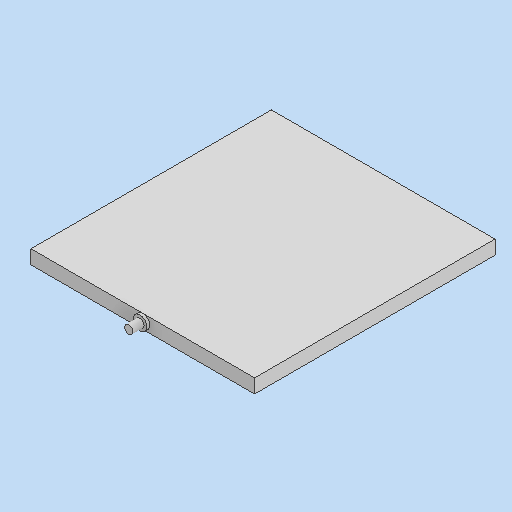
# Autodesk Inventor part: brush
Saved by Autodesk Inventor 2026 (Build 300175000, 175)
## iProperties
Created: 2026-02-15
Part Number: brush
Material: Generic
Document SubType Name: Modeling
Designer: mones
Density: 1 g/cm^3
Appearance: Default
Author: mones
Autodesk Inventor part; units mm, degrees
ref_plane "YZ Plane" through (0, 0, 0) normal (1, 0, 0) x (0, 1, 0)
ref_plane "XZ Plane" through (0, 0, 0) normal (0, 1, 0) x (-1, 0, 0)
ref_plane "XY Plane" through (0, 0, 0) normal (0, 0, 1) x (1, 0, 0)
sketch "Sketch1" plane through (0, 0, 0) normal (0, 1, 0) x (-1, 0, 0)
  line L0 (40, 43) -> (40, -43)
  line L1 (40, -43) -> (-40, -43)
  line L2 (-40, -43) -> (-40, 43)
  line L3 (-40, 43) -> (40, 43)
  line L4 (40, 43) -> (-40, -43) construction
  line L5 (40, -43) -> (-40, 43) construction
  point P0 (0, 0)
  dimension "d0" = 86
  dimension "d1" = 80
  constraints: 12 end point, 2 midpoint, 2 parallel, 1 perpendicular, 1 vertical
  measures "d0" distance of L0.start L0.end
  measures "d1" distance of L0.end L1.end
extrude "Extrusion1" add sketch "Sketch1" along normal blind 5
sketch "Sketch2" plane through (40, 0, -43) normal (0, 0, -1) x (-1, 0, 0)
  line L0 (0, 0) -> (80, 0) projected
  line L1 (80, 0) -> (80, 5) projected
  line L2 (0, 5) -> (80, 5) projected
  line L3 (0, 0) -> (0, 5) projected
  circle A0 centre (40.1562, 2.5) radius 1.5
  dimension "d4" = 3
  constraints: 1 centre point
  measures "d4" diameter of A0
extrude "Extrusion2" cut sketch "Sketch2" against normal blind 6 contours A0
sketch "Sketch3" plane through (-40, 0, 43) normal (0, 0, 1) x (1, 0, 0)
  line L0 (0, 0) -> (80, 0) projected
  line L1 (80, 0) -> (80, 5) projected
  line L2 (0, 5) -> (80, 5) projected
  line L3 (0, 0) -> (0, 5) projected
  circle A0 centre (40, 2.5) radius 2.5
  dimension "d7" = 5
  constraints: 1 centre point
  measures "d7" diameter of A0
extrude "Extrusion3" add sketch "Sketch3" along normal blind 1 contours A0
sketch "Sketch4" plane through (0, 2.5, 44) normal (0, 0, 1) x (1, 0, 0)
  circle A0 centre (0, 0) radius 1.5
  dimension "d10" = 3
  constraints: 1 centre point
  measures "d10" diameter of A0
extrude "Extrusion4" add sketch "Sketch4" along normal blind 4
body "Solid1"
